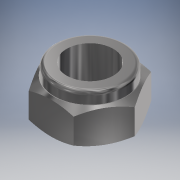
# Autodesk Inventor part: M6 K-Nut Short
Saved by Autodesk Inventor 2019 (Build 230136000, 136)
## iProperties
Created: 2007-11-24
Part Number: M6 K-Nut Short
Document SubType Name: Modeling
Designer: Administrator
Material: Steel
Density: 7.85 g/cm^3
Appearance: Stainless - Brushed
Description: Plain M6 K-Nut
Author: Administrator
Autodesk Inventor part; units mm, degrees
ref_plane "YZ Plane" through (0, 0, 0) normal (1, 0, 0) x (0, 1, 0)
ref_plane "XZ Plane" through (0, 0, 0) normal (0, 1, 0) x (-1, 0, 0)
ref_plane "XY Plane" through (0, 0, 0) normal (0, 0, 1) x (1, 0, 0)
sketch "Sketch1" plane through (0, 0, 0) normal (0, 0, 1) x (1, 0, 0)
  circle A0 centre (0, 0) radius 3
  line L0 (-2.8868, 5) -> (2.8868, 5)
  line L1 (2.8868, 5) -> (5.7735, 0)
  line L2 (5.7735, 0) -> (2.8868, -5)
  line L3 (2.8868, -5) -> (-2.8868, -5)
  line L4 (-2.8868, -5) -> (-5.7735, 0)
  line L5 (-5.7735, 0) -> (-2.8868, 5)
  dimension "d0" = 6
  dimension "d1" = 10
  constraints: 12 end point, 2 coincident, 1 centre point, 1 horizontal, 13 other
  measures "d0" diameter of A0
  measures "d1" distance between parallel lines of L3 L0
extrude "Extrusion1" add sketch "Sketch1" along normal mid plane 4.5
sketch "Sketch2" plane through (0, 0, 2.25) normal (0, 0, 1) x (1, 0, 0)
  circle A0 centre (0, 0) radius 3 projected
  circle A1 centre (0, 0) radius 4.6
  dimension "d6" = 9.2
  constraints: 1 centre point, 1 coincident
  measures "d6" diameter of A1
extrude "Extrusion2" add sketch "Sketch2" along normal blind 1.5
sketch "Sketch4" plane through (0, 0, 0) normal (0, 1, 0) x (-1, 0, 0)
  line L0 (-2.8868, 2.25) -> (-5.7735, 2.25) projected
  line L1 (-5.7735, 2.25) -> (-5.7735, -2.25) projected
  line L2 (-5.7735, -2.25) -> (-2.8868, -2.25) projected
  line L3 (-2.8868, 2.25) -> (-2.8868, -2.25) projected
  line L4 (-4.6735, 2.25) -> (-5.7735, 1.6149)
  line L5 (-5.7735, -1.6149) -> (-4.6735, -2.25)
  line L6 (0, -3.5) -> (0, 3.5) projected
  dimension "d7" = 1.1
  dimension "d8" = 1.1
  dimension "d9" = 30
  dimension "d10" = 30
  constraints: 4 end point, 4 point on line
  measures "d7" horizontal distance of L4.end L4.start
  measures "d8" distance from line of L1 L5.end
  measures "d9" angle of L0 L4
  measures "d10" angle of L2 L5
revolve "Revolution1" cut sketch "Sketch4" angle 360 about axis through (0, 0, -10) along (0, 0, 1) contours L4 L1 L0 | L2 L1 L5
fillet "Fillet1" radius 0.5 1 edges at (-4.6, 0, 3.75)
body "Solid1"
